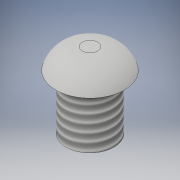
# Autodesk Inventor part: screwLarge
Saved by Autodesk Inventor 2019.1 (Build 231200000, 200)
## iProperties
Created: 2018-12-04
Part Number: screwLarge
Material: Generic
Document SubType Name: Modeling
Designer: kfortuna
Density: 1 g/cm^3
Appearance: Default
Author: kfortuna
Autodesk Inventor part; units mm, degrees
ref_plane "YZ Plane" through (0, 0, 0) normal (1, 0, 0) x (0, 1, 0)
ref_plane "XZ Plane" through (0, 0, 0) normal (0, 1, 0) x (-1, 0, 0)
ref_plane "XY Plane" through (0, 0, 0) normal (0, 0, 1) x (1, 0, 0)
sketch "Sketch1" plane through (0, 0, 0) normal (0, 1, 0) x (-1, 0, 0)
  circle A0 centre (25.8401, 17.3142) radius 1.75
  point P0 (0, 0)
  dimension "d0" = 3.5
  constraints: 1 centre point
  measures "d0" diameter of A0
extrude "Extrusion1" add sketch "Sketch1" along normal blind 4
thread "Thread1" size "M3.5x0.6" class "6g" standard "ANSI Metric M Profile" full length
sketch "Sketch2" plane through (-25.8401, 4, 17.3142) normal (0, 1, 0) x (1, 0, 0)
  circle A0 centre (0, 0) radius 2.5
  point P0 (25.8401, 17.3142)
  dimension "d5" = 5
  constraints: 1 centre point
  measures "d5" diameter of A0
extrude "Extrusion2" add sketch "Sketch2" along normal blind 1.5
fillet "Fillet1" radius 2 1 edges at (-28.3401, 5.5, 17.3142)
body "Solid1"
